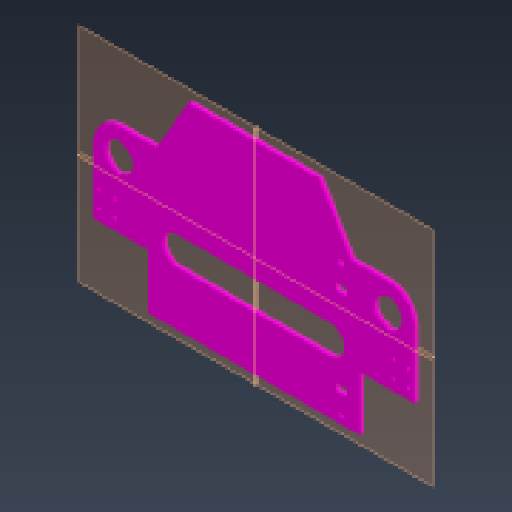
# Autodesk Inventor part: Передняя_крышка
Saved by Autodesk Inventor 2023.2 (Build 272271030, 271C)
## iProperties
Created: 2025-12-12
Part Number: Передняя_крышка
Material: Типовые
Document SubType Name: Modeling
Designer: Олег Коноваленко
Density: 1 g/cm^3
Appearance: Пурпурный
Author: Олег Коноваленко
Autodesk Inventor part; units mm, degrees
sketch "Эскиз1" plane through (0, 0, 0) normal (0, 0, 1) x (1, 0, 0)
  line L0 (-147, -42.5) -> (147, -42.5)
  line L1 (147, -42.5) -> (147, 42.5)
  line L2 (147, 42.5) -> (-147, 42.5)
  line L3 (-147, 42.5) -> (-147, -42.5)
  line L4 (-147, -42.5) -> (147, 42.5) construction
  line L5 (147, -42.5) -> (-147, 42.5) construction
  point P0 (0, 0)
  dimension "d0" = 294
  dimension "d1" = 85
  constraints: 12 end point, 2 midpoint, 2 parallel, 1 horizontal, 1 perpendicular
  measures "d0" distance of L1.end L2.end
  measures "d1" distance of L2.end L0.start
extrude "Выдавливание1" add sketch "Эскиз1" along normal mid plane 4
sketch "Эскиз5" plane through (0, 0, 2) normal (0, 0, 1) x (1, 0, 0)
  arc A0 (147, 17.5) -> (122, 42.5) centre (122, 17.5) ccw projected
  line L0 (147, -42.5) -> (147, 42.5) projected
  line L1 (147, 42.5) -> (-147, 42.5) projected
  point P0 (0, 0)
  point P1 (147, 17.5)
extrude "Выдавливание4" cut sketch "Эскиз5" against normal up to next
sketch "Эскиз6" plane through (0, 0, -2) normal (0, 0, -1) x (-1, 0, 0)
  line L0 (147, -42.5) -> (-147, -42.5) projected
  line L1 (-97, -42.5) -> (97, -42.5)
  line L2 (97, -42.5) -> (97, -92.5)
  line L3 (97, -92.5) -> (-97, -92.5)
  line L4 (-97, -92.5) -> (-97, -42.5)
  line L5 (-97, -92.5) -> (-97, -42.5) projected
  line L6 (147, -42.5) -> (147, 42.5) projected
  point P0 (0, 0)
  dimension "d18" = 50
  constraints: 8 end point, 2 parallel, 1 horizontal, 1 perpendicular, 1 point on line
  measures "d18" distance between parallel lines of L6 L2
extrude "Выдавливание5" add sketch "Эскиз6" against normal blind 4
sketch "Эскиз7" plane through (0, 0, -2) normal (0, 0, -1) x (-1, 0, 0)
  circle A0 centre (-127.5, -32.5) radius 1.6 projected
  circle A1 centre (-127.5, -17.5) radius 1.6 projected
  circle A2 centre (-141.5, -17.5) radius 1.6 projected
  circle A3 centre (-141.5, -32.5) radius 1.6 projected
  point P0 (0, 0)
extrude "Выдавливание6" cut sketch "Эскиз7" against normal up to next
sketch "Эскиз8" plane through (0, 0, -2) normal (0, 0, -1) x (-1, 0, 0)
  circle A0 centre (-122, 17.5) radius 6 projected
  circle A1 centre (-122, 17.5) radius 13.5
  point P0 (0, 0)
  dimension "d23" = 7.5
  constraints: 1 centre point
  measures "d23" radial gap between concentric circles of A1 A0
extrude "Выдавливание7" cut sketch "Эскиз8" against normal up to next contours A0 | A1
sketch "Эскиз9" plane through (0, 0, -2) normal (0, 0, -1) x (-1, 0, 0)
  circle A0 centre (-122, 17.5) radius 13.5 projected
  arc A1 (-122, 6) -> (-122, 29) centre (-122, 17.5) ccw
  line L0 (-122, 4) -> (-122, 31)
  point P0 (0, 0)
  dimension "d26" = 11.5
  constraints: 4 point on circle, 2 end point, 2 point on line, 1 centre point, 1 concentric, 1 midpoint, 1 vertical
  measures "d26" radius of A1
extrude "Выдавливание8" add sketch "Эскиз9" against normal blind 4 contours A0 L0 A1
mirror "Зеркальное отражение1" about plane through (0, 0, 0) normal (1, 0, 0) of "Выдавливание6", "Выдавливание7", "Выдавливание8", "Выдавливание4"
fillet "Сопряжение2" radius 3 4 edges at (122, 6, 0) (122, 29, 0) (-122, 29, 0) (-122, 6, 0)
sketch "Эскиз10" plane through (0, 0, -2) normal (0, 0, -1) x (-1, 0, 0)
  line L0 (70, -30) -> (-70, -30) construction
  line L1 (70, -17) -> (-70, -17)
  line L2 (-70, -43) -> (70, -43)
  arc A0 (70, -43) -> (70, -17) centre (70, -30) ccw
  arc A1 (-70, -17) -> (-70, -43) centre (-70, -30) ccw
  line L3 (0, -119.5) -> (0, 69.5) projected
  line L4 (-205.8, 0) -> (205.8, 0) projected
  point P0 (0, 0)
  point P1 (0, -30)
  dimension "d32" = 140
  dimension "d33" = 30
  dimension "d34" = 13
  constraints: 8 end point, 4 point on circle, 4 tangent, 2 centre point, 1 horizontal, 1 midpoint, 1 parallel, 1 point on line
  measures "d32" distance of L0.start L0.end
  measures "d33" distance between parallel lines of L4 L0
  measures "d34" distance between parallel lines of L0 L2
extrude "Выдавливание9" cut sketch "Эскиз10" against normal up to next
sketch "Эскиз11" plane through (0, 0, -2) normal (0, 0, -1) x (-1, 0, 0)
  circle A0 centre (-80, -85.5) radius 1.79 projected
  line L0 (-85.2, -61.87) -> (-74.8, -61.87) projected
  line L1 (-74.8, -61.87) -> (-74.8, -67.77) projected
  line L2 (-74.8, -67.77) -> (-85.2, -67.77) projected
  line L3 (-85.2, -67.77) -> (-85.2, -61.87) projected
  circle A1 centre (-80, 35.5) radius 2.5 projected
  line L4 (-74.8, 11.87) -> (-85.2, 11.87) projected
  line L5 (-74.8, 17.77) -> (-74.8, 11.87) projected
  line L6 (-85.2, 17.77) -> (-74.8, 17.77) projected
  line L7 (-85.2, 17.77) -> (-85.2, 11.87) projected
  point P0 (0, 0)
extrude "Выдавливание10" cut sketch "Эскиз11" against normal up to next
sketch "Эскиз12" plane through (0, 0, -2) normal (0, 0, -1) x (-1, 0, 0)
  line L0 (-122, 42.5) -> (122, 42.5) projected
  line L1 (88.8675, 42.5) -> (60, 92.5)
  line L2 (60, 92.5) -> (-60, 92.5)
  line L3 (-60, 92.5) -> (-88.8675, 42.5)
  line L4 (0, -129.6087) -> (0, 130.1524) construction
  point P0 (0, 0)
  point P1 (0, 92.5)
  dimension "d39" = 120
  dimension "d40" = 50
  dimension "d41" = 120
  dimension "d42" = 120
  constraints: 6 end point, 3 point on line, 1 midpoint, 1 parallel
  measures "d39" distance of L1.end L2.end
  measures "d40" distance between parallel lines of L0 L2
  measures "d41" angle of L1 L2
  measures "d42" angle of L2 L3
extrude "Выдавливание11" add sketch "Эскиз12" against normal blind 4
